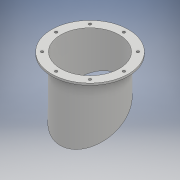
# Autodesk Inventor part: 进气孔
Saved by Autodesk Inventor 2018.2 (Build 222227000, 227)
## iProperties
Created: 2018-07-04
Part Number: 进气孔
Material: 常规
Document SubType Name: Modeling
Designer: Administrator
Density: 1 g/cm^3
Appearance: 默认
Author: Administrator
Autodesk Inventor part; units mm, degrees
ref_plane "YZ Plane" through (0, 0, 0) normal (1, 0, 0) x (0, 1, 0)
ref_plane "XZ Plane" through (0, 0, 0) normal (0, 1, 0) x (-1, 0, 0)
ref_plane "XY Plane" through (0, 0, 0) normal (0, 0, 1) x (1, 0, 0)
sketch "草图1" plane through (0, 0, 0) normal (0, 0, 1) x (1, 0, 0)
  circle A0 centre (0, 0) radius 225
  dimension "d0" = 450
  constraints: 1 centre point, 1 coincident
  measures "d0" diameter of A0
surface extrude "拉伸曲面1" sketch "草图1" along normal blind 500 shown no curves A0
thicken "加厚1" operation new thickness 3.7 both sides no extend neighbours no toward (-0.4864037, 0.8737342, 0) faces at (109.4408, -196.5902, 333.3333)
sketch "草图2" plane through (0, 0, 500) normal (0, 0, 1) x (1, 0, 0)
  circle A0 centre (0, 0) radius 225 projected
  circle A1 centre (0, 0) radius 221.3 projected
  circle A2 centre (0, 0) radius 290
  dimension "d18" = 580
  dimension "d19" = 442.6
  dimension "d20" = 450
  constraints: 1 centre point, 1 coincident
  measures "d18" diameter of A2
  measures "d19" diameter of A1
  measures "d20" diameter of A0
extrude "拉伸1" add sketch "草图2" against normal blind 15 contours A2
sketch "草图3" plane through (0, 0, 500) normal (0, 0, 1) x (1, 0, 0)
  circle A0 centre (0, 0) radius 290 projected
  circle A1 centre (0, 0) radius 221.3 projected
  line L0 (0, -221.3) -> (0, -290)
  point P0 (0, -255.65)
  point P1 (180.7718, -180.7718)
  point P2 (255.65, 0)
  point P3 (180.7718, 180.7718)
  point P4 (0, 255.65)
  point P5 (-180.7718, 180.7718)
  point P6 (-255.65, 0)
  point P7 (-180.7718, -180.7718)
  dimension "d9" = 360
  dimension "d21" = 255.65
  constraints: 2 end point, 2 vertical alignment, 1 midpoint, 11 other
  measures "d21" distance of point (-255.65, 0) point (0, 0)
hole "孔1" at (0, -255.65, 500) at (180.7718, -180.7718, 500) at (255.65, 0, 500) at (180.7718, 180.7718, 500) at (0, 255.65, 500) at (-180.7718, 180.7718, 500) at (-255.65, 0, 500) at (-180.7718, -180.7718, 500) direction (0, 0, -1) diameter 20 end through all
sketch "草图4" plane through (0, 0, 0) normal (1, 0, 0) x (0, 1, 0)
  line L0 (-225, 485) -> (225, 485) projected
  line L1 (225, 0) -> (-225, 0) projected
  line L2 (225, 0) -> (-225, 0) projected
  line L3 (-225, 0) -> (225, 242.5)
  line L4 (225, 0) -> (225, 485) projected
  point P0 (0, 0)
  constraints: 2 end point, 1 midpoint
extrude "拉伸2" cut sketch "草图4" along normal mid plane 1000
body "Srf1"
